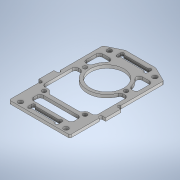
# Autodesk Inventor part: 胴体_サブフレーム_仮１
Saved by Autodesk Inventor 2020.4 (Build 244396000, 396)
## iProperties
Created: 2021-09-09
Part Number: 胴体_サブフレーム_仮１
Material: 一般
Document SubType Name: Modeling
Designer: moonk
Density: 1 g/cm^3
Appearance: 既定
Author: moonk
Autodesk Inventor part; units mm, degrees
ref_plane "YZ Plane" through (0, 0, 0) normal (1, 0, 0) x (0, 1, 0)
ref_plane "XZ Plane" through (0, 0, 0) normal (0, 1, 0) x (-1, 0, 0)
ref_plane "XY Plane" through (0, 0, 0) normal (0, 0, 1) x (1, 0, 0)
sketch "スケッチ1" plane through (0, 0, 0) normal (0, 0, 1) x (1, 0, 0)
  circle A0 centre (0, 0) radius 11
  line L0 (-10, 22) -> (10, 22)
  line L1 (17.75, -44.5) -> (-17.75, -44.5)
  line L2 (-15, 16.5) -> (15, 16.5) construction
  line L3 (15, 16.5) -> (15, -42) construction
  line L4 (15, -42) -> (-15, -42) construction
  line L5 (-15, -42) -> (-15, 16.5) construction
  circle A1 centre (-15, 16.5) radius 1.55
  circle A2 centre (15, 16.5) radius 1.55
  circle A3 centre (-15, -42) radius 1.55
  circle A4 centre (15, -42) radius 1.55
  line L6 (-17.75, -44.5) -> (-20, -44.5)
  line L7 (-20, -44.5) -> (-20, 17.12)
  line L8 (-10, 22) -> (-20, 17.12)
  line L9 (0, 22) -> (0, -44.5) construction
  line L10 (-20, -23) -> (-22, -23)
  line L11 (-22, -23) -> (-22, -13)
  line L12 (-22, -13) -> (-20, -13)
  line L13 (17.75, -44.5) -> (20, -44.5)
  line L14 (20, -44.5) -> (20, 17.12)
  line L15 (10, 22) -> (20, 17.12)
  line L16 (20, -23) -> (22, -23)
  line L17 (22, -23) -> (22, -13)
  line L18 (22, -13) -> (20, -13)
  line L19 (13.5, -1) -> (-13.5, -1) construction
  line L20 (-13.5, -1) -> (-13.5, -28) construction
  line L21 (-13.5, -28) -> (13.5, -28) construction
  line L22 (13.5, -28) -> (13.5, -1) construction
  circle A5 centre (-13.5, -1) radius 1.35
  circle A6 centre (-13.5, -28) radius 1.35
  circle A7 centre (13.5, -1) radius 1.35
  circle A8 centre (13.5, -28) radius 1.35
  line L23 (10.01, -42) -> (-10.01, -42)
  line L24 (-10.01, -42) -> (-10.01, -39.48)
  line L25 (-10.01, -39.48) -> (10.01, -39.48)
  line L26 (10.01, -39.48) -> (10.01, -42)
  circle A9 centre (-8.96, -39.48) radius 1.05
  circle A10 centre (-8.96, -42) radius 1.05
  circle A11 centre (8.96, -42) radius 1.05
  circle A12 centre (8.96, -39.48) radius 1.05
  line L27 (-10.1, 19.01) -> (10.1, 19.01)
  line L28 (10.1, 19.01) -> (10.1, 16.49)
  line L29 (10.1, 16.49) -> (-10.1, 16.49)
  line L30 (-10.1, 16.49) -> (-10.1, 19.01)
  circle A13 centre (-9.05, 19.01) radius 1.05
  circle A14 centre (-9.05, 16.49) radius 1.05
  circle A15 centre (9.05, 16.49) radius 1.05
  circle A16 centre (9.05, 19.01) radius 1.05
  arc A17 (-20, -25.1) -> (-20, -23) centre (-20, -24.05) ccw
  arc A18 (-20, -13) -> (-20, -10.9) centre (-20, -11.95) ccw
  arc A19 (20, -23) -> (20, -25.1) centre (20, -24.05) ccw
  arc A20 (20, -10.9) -> (20, -13) centre (20, -11.95) ccw
  point P0 (7.91, -42)
  point P1 (-7.91, -42)
  point P2 (-7.91, -39.48)
  point P3 (7.91, -39.48)
  point P4 (8, 16.49)
  point P5 (-8, 16.49)
  point P6 (-10.1, 19.01)
  point P7 (-8, 19.01)
  point P8 (8, 19.01)
  point P9 (0, -39.48)
  point P10 (0, 16.49)
  point P11 (0, 19.01)
  point P12 (20, -25.1)
  dimension "d111" = 2.1
  dimension "d140" = 2.1
  dimension "d141" = 2.1
  dimension "d147" = 2.1
  dimension "d0" = 22
  dimension "d1" = 20
  dimension "d3" = 35.5
  dimension "d6" = 44.5
  dimension "d12" = 66.5
  dimension "d21" = 58.5
  dimension "d23" = 5.5
  dimension "d25" = 3.1
  dimension "d26" = 3.1
  dimension "d27" = 3.1
  dimension "d28" = 3.1
  dimension "d38" = 2
  dimension "d39" = 10
  dimension "d42" = 15
  dimension "d43" = 30
  dimension "d44" = 35
  dimension "d45" = 15
  dimension "d62" = 27
  dimension "d63" = 27
  dimension "d64" = 13.5
  dimension "d65" = 1
  dimension "d66" = 2.7
  dimension "d67" = 2.7
  dimension "d68" = 2.7
  dimension "d69" = 2.7
  dimension "d104" = 20.02
  dimension "d105" = 2.52
  dimension "d109" = 2.1
  dimension "d110" = 2.1
  dimension "d112" = 2.1
  dimension "d129" = 16.5
  dimension "d131" = 39.48
  dimension "d133" = 2.52
  dimension "d134" = 20.2
  dimension "d136" = 5.51
  dimension "d139" = 2.1
  dimension "d149" = 40
  dimension "d150" = 2.75
  dimension "d151" = 1.05
  dimension "d152" = 1.05
  constraints: 62 end point, 20 point on line, 17 centre point, 10 parallel, 10 symmetric about line, 9 coincident, 8 point on circle, 7 horizontal, 6 perpendicular, 5 midpoint, 4 tangent, 2 vertical, 14 other
  measures "d0" diameter of A0
  measures "d1" distance of L0.start L0.end
  measures "d3" distance of L1.start L1.end
  measures "d6" distance from line of L1 point (0, 0)
  measures "d12" distance between parallel lines of L0 L1
  measures "d21" distance of L2.end L3.end
  measures "d23" distance between parallel lines of L2 L0
  measures "d25" diameter of A1
  measures "d26" diameter of A2
  measures "d27" diameter of A3
  measures "d28" diameter of A4
  measures "d38" distance of L10.start L10.end
  measures "d39" distance of L10.end L11.end
  measures "d42" distance between parallel lines of L3 L9
  measures "d43" distance between parallel lines of L5 L3
  measures "d44" distance between parallel lines of L12 L0
  measures "d45" distance from line of point (0, 0) L3
  measures "d62" distance of L21.end L20.end
  measures "d63" distance of L20.end L19.end
  measures "d64" distance between parallel lines of L9 L20
  measures "d65" distance from line of L19 A0.centre
  measures "d66" diameter of A5
  measures "d67" diameter of A6
  measures "d68" diameter of A7
  measures "d69" diameter of A8
  measures "d104" distance of L24.end L25.end
  measures "d105" distance of L23.end L24.end
  measures "d109" diameter of A9
  measures "d110" diameter of A10
  measures "d112" diameter of A12
  measures "d129" distance from line of point (0, 0) L2
  measures "d131" distance from line of L25 point (0, 0)
  measures "d133" distance of L27.end L28.end
  measures "d134" distance between parallel lines of L28 L30
  measures "d136" distance between parallel lines of L29 L0
  measures "d139" diameter of A13
  measures "d149" distance of L6.end L14.start
  measures "d150" distance from line of A1.centre L8
  measures "d151" radius of A17
  measures "d152" radius of A18
extrude "押し出し1" add sketch "スケッチ1" along normal blind 2 contours L0 L15 L14 A20 A19 L13 L1 L6 L7 A17 A18 L8 | L7 L10 L11 L12 | L18 L17 L16 L14
sketch "スケッチ2" plane through (0, 0, 2) normal (0, 0, 1) x (1, 0, 0)
  circle A0 centre (-13.5, -28) radius 1.35 projected
  circle A1 centre (13.5, -28) radius 1.35 projected
  circle A2 centre (-13.5, -1) radius 1.35 projected
  circle A3 centre (13.5, -1) radius 1.35 projected
  circle A4 centre (0, 0) radius 13 construction
  line L0 (20, -44.5) -> (20, 17.12) projected
  line L1 (-20, 17.12) -> (-20, -44.5) projected
  line L2 (10, 22) -> (-10, 22) projected
  line L3 (0, 22) -> (0, -44.5) construction
  line L4 (-20, -44.5) -> (20, -44.5) projected
  circle A5 centre (-13.5, -1) radius 2.6 construction
  circle A6 centre (13.5, -1) radius 2.6 construction
  circle A7 centre (-13.5, -28) radius 2.6 construction
  circle A8 centre (13.5, -28) radius 2.6 construction
  arc A9 (-3.8182, 12.4266) -> (-12.8912, 1.6787) centre (0, 0) ccw
  arc A10 (12.8912, 1.6787) -> (3.8182, 12.4266) centre (0, 0) ccw
  arc A11 (-12.4916, -3.6) -> (12.4916, -3.6) centre (0, 0) ccw
  arc A12 (-10.9, -28) -> (-13.5, -25.4) centre (-13.5, -28) ccw
  arc A13 (13.5, -25.4) -> (10.9, -28) centre (13.5, -28) ccw
  line L5 (-10.9, -28) -> (10.9, -28)
  line L6 (-13.4907, -30.6) -> (13.5093, -30.6)
  arc A14 (-7.91, -39.48) -> (-10.01, -39.48) centre (-8.96, -39.48) ccw projected
  circle A15 centre (-8.96, -39.48) radius 2.45 construction
  arc A16 (10.01, -39.48) -> (7.91, -39.48) centre (8.96, -39.48) ccw projected
  circle A17 centre (8.96, -39.48) radius 2.45 construction
  line L7 (-13.4907, -30.6) -> (-13.4907, -37.03)
  line L8 (-13.4907, -37.03) -> (13.5093, -37.03)
  line L9 (13.5093, -37.03) -> (13.5093, -30.6)
  line L10 (-17.5, 12.5022) -> (-3.8182, 12.4266)
  line L11 (-17.5, 12.5022) -> (-17.5, 1.6787)
  line L12 (-17.5, 1.6787) -> (-12.8912, 1.6787)
  arc A18 (12.8912, 1.6787) -> (3.8182, 12.4266) centre (0, 0) ccw
  line L13 (17.5, 12.5022) -> (3.8182, 12.4266)
  line L14 (17.5, 12.5022) -> (17.5, 1.6787)
  line L15 (17.5, 1.6787) -> (12.8912, 1.6787)
  line L16 (-17.48, -3.6) -> (-12.4916, -3.6)
  line L17 (-17.48, -3.6) -> (-17.48, -25.4)
  line L18 (-17.48, -25.4) -> (-13.5, -25.4)
  line L19 (17.5, -3.6) -> (12.4916, -3.6)
  line L20 (17.5, -3.6) -> (17.5, -25.4)
  line L21 (17.5, -25.4) -> (13.5, -25.4)
  dimension "d76" = 26
  dimension "d82" = 5.2
  dimension "d83" = 5.2
  dimension "d84" = 5.2
  dimension "d85" = 5.2
  dimension "d88" = 23.8182
  dimension "d89" = 32.8912
  dimension "d92" = 21.8
  dimension "d94" = 13
  dimension "d115" = 4.9
  dimension "d116" = 4.9
  dimension "d117" = 6.5093
  dimension "d118" = 7.47
  dimension "d123" = 10.8236
  dimension "d124" = 2.5
  dimension "d125" = 21.8
  dimension "d126" = 34.98
  dimension "d127" = 2.5
  constraints: 36 end point, 22 point on circle, 13 centre point, 7 coincident, 5 perpendicular, 4 symmetric about line, 3 concentric, 3 horizontal, 3 vertical, 2 midpoint, 2 point on line, 2 tangent, 1 parallel, 2 other
  measures "d76" diameter of A4
  measures "d82" diameter of A5
  measures "d83" diameter of A6
  measures "d84" diameter of A7
  measures "d85" diameter of A8
  measures "d88" distance from line of L10.end L0
  measures "d89" distance from line of L12.end L0
  measures "d92" distance of L5.start L5.end
  measures "d94" radius of A11
  measures "d115" diameter of A15
  measures "d116" diameter of A17
  measures "d117" distance between parallel lines of L7 L1
  measures "d118" distance between parallel lines of L4 L8
  measures "d123" distance of L10.start L11.end
  measures "d124" distance between parallel lines of L1 L11
  measures "d125" distance of L16.start L17.end
  measures "d126" distance between parallel lines of L17 L20
  measures "d127" distance between parallel lines of L20 L0
extrude "押し出し2" cut sketch "スケッチ2" against normal blind 2 contours A9 L12 L11 L10 | A10 L13 L14 L15 | A11 L19 L20 L21 A13 L5 A12 L18 L17 L16 | L6 L9 L8 L7
fillet "フィレット2" radius 2 20 edges at (-17.5, 12.5022, 1) (-3.8182, 12.4266, 1) (17.5, 12.5022, 1) (-12.8912, 1.6787, 1) (17.5, 1.6787, 1) (3.8182, 12.4266, 1) (-17.5, 1.6787, 1) (12.8912, 1.6787, 1) (17.5, -3.6, 1) (12.4916, -3.6, 1) (-12.4916, -3.6, 1) (-17.48, -3.6, 1) (-17.48, -25.4, 1) (-10.9, -28, 1) (17.5, -25.4, 1) (10.9, -28, 1) (13.5093, -37.03, 1) (-13.4907, -37.03, 1) (-13.4907, -30.6, 1) (13.5093, -30.6, 1)
fillet "フィレット3" radius 1 6 edges at (-20, -44.5, 1) (20, -44.5, 1) (-20, 17.12, 1) (-10, 22, 1) (10, 22, 1) (20, 17.12, 1)
equation "\"d26\" = d25"
equation "\"d27\" = d25"
equation "\"d28\" = d25"
equation "\"d67\" = d66"
equation "\"d68\" = d66"
equation "\"d69\" = d66"
